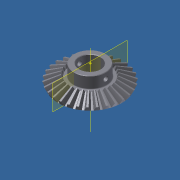
# Autodesk Inventor part: Bevel Gear1
Saved by Autodesk Inventor 2012 SP2 (Build 160219200, 219)
## iProperties
Created: 2012-07-24
Part Number: Bevel Gear1
Material: Steel, Mild
Document SubType Name: Modeling
Designer: bruno.silveira
Categories: <?xml version="1.0" encoding="UTF-16"?> <MemberInstance><Categories><FamilyTemplate><FamilyTemplateParameter ValueType="xs:double" Id="1" ObjectReferenceKey="da_z" ObjectType="kUserParameterObject"/><FamilyTemplateParameter ValueType="xs:double" Id="2" ObjectReferenceKey="da_b" ObjectType="kUserParameterObject"/><FamilyTemplateParameter ValueType="xs:double" Id="3" ObjectReferenceKey="da_beta" ObjectType="kUserParameterObject"/><FamilyTemplateParameter ValueType="xs:double" Id="4" ObjectReferenceKey="da_dae" ObjectType="kUserParameterObject"/><FamilyTemplateParameter ValueType="xs:double" Id="5" ObjectReferenceKey="da_ve" ObjectType="kUserParameterObject"/><FamilyTemplateParameter ValueType="xs:double" Id="6" ObjectReferenceKey="da_omega" ObjectType="kUserParameterObject"/><FamilyTemplateParameter ValueType="xs:string" Id="7" ObjectReferenceKey="EAIAABAAAAAAHwAAAAAAAIAAAAAAAAAA" ObjectType="83914240" SubObjectId="SurfaceGeometry"/></FamilyTemplate><ParamToTemplateMap><ParamToTemplate CategoryParameter="//CategoryParameter[@InternalName='046C89C9-8512-4d59-83FE-43B91F4F132A']" TemplateParameter="1"/><ParamToTemplate CategoryParameter="//CategoryParameter[@InternalName='2552DF32-E462-4b46-AEBF-C6C7768E72AC']" TemplateParameter="2"/><ParamToTemplate CategoryParameter="//CategoryParameter[@InternalName='C9EE641D-15FC-4fae-A226-E94C4372FDD7']" TemplateParameter="3"/><ParamToTemplate><ParamToTemplate CategoryParameter="//CategoryParameter[@InternalName='00B6519A-459B-49c7-AD84-2E56D39A5744']" ConstantValue="0.000000"/></ParamToTemplate><ParamToTemplate><ParamToTemplate CategoryParameter="//CategoryParameter[@InternalName='04B31F0E-C7A6-4894-AA32-9629BEFACF47']" ConstantValue="1.000000"/></ParamToTemplate><ParamToTemplate><ParamToTemplate CategoryParameter="//CategoryParameter[@InternalName='43CBEC2E-7847-49e7-A936-2F7889FCB2D9']" ConstantValue="0.200000"/></ParamToTemplate><ParamToTemplate><ParamToTemplate CategoryParameter="//CategoryParameter[@InternalName='B1EFC894-105D-4ebd-86BF-FA20ED196853']" ConstantValue="0.300000"/></ParamToTemplate><ParamToTemplate><ParamToTemplate CategoryParameter="//CategoryParameter[@InternalName='51175063-3D10-4879-93E8-6246FE8B403D']" ConstantValue="2060000000.000000"/></ParamToTemplate><ParamToTemplate><ParamToTemplate CategoryParameter="//CategoryParameter[@InternalName='A3A52E27-4454-46a9-B0BD-C932399B70AF']" ConstantValue="0.300000"/></ParamToTemplate><ParamToTemplate CategoryParameter="//CategoryParameter[@InternalName='2A200944-5A8C-41ca-B96E-8520D2E510F1']" TemplateParameter="4"/><ParamToTemplate><ParamToTemplate CategoryParameter="//CategoryParameter[@InternalName='1A637F62-92C8-44bc-B81F-10802510B579']" ConstantValue="2.791976"/></ParamToTemplate><ParamToTemplate CategoryParameter="//CategoryParameter[@InternalName='B52DD4BE-6863-48fb-BF58-89EF6F9EC65C']" TemplateParameter="5"/><ParamToTemplate><ParamToTemplate CategoryParameter="//CategoryParameter[@InternalName='3956BFF2-84D2-457d-93C2-9B0613DEBA67']" ConstantValue="0.596956"/></ParamToTemplate><ParamToTemplate CategoryParameter="//CategoryParameter[@InternalName='739CFA02-461B-4bf8-8049-181FCAD8B28F']" TemplateParameter="6"/><ParamToTemplate><ParamToTemplate CategoryParameter="//CategoryParameter[@InternalName='A27E999F-E2CE-4481-8A2A-EBF499C4C3C5']" ConstantValue="0.000000"/></ParamToTemplate><ParamToTemplate><ParamToTemplate CategoryParameter="//CategoryParameter[@InternalName='9E1B4470-B2D3-4ff1-B813-535BB4CDF51A']" ConstantValue="3520000.000000"/></ParamToTemplate><ParamToTemplate><ParamToTemplate CategoryParameter="//CategoryParameter[@InternalName='F8452263-BFF6-458c-9FB1-07C4B99E95CD']" ConstantValue="11400000.000000"/></ParamToTemplate><ParamToTemplate><ParamToTemplate CategoryParameter="//CategoryParameter[@InternalName='3E3BB259-FD49-497f-8171-6EBC954A3479']" ConstantValue="2.000000"/></ParamToTemplate><ParamToTemplate CategoryParameter="//CategoryParameter[@InternalName='27C3BAF2-7550-4e4b-AE2C-0DB134B7D9B7']" TemplateParameter="7"/></ParamToTemplateMap><Category DisplayName="Gear" InternalName="DC85795E-93AB-48d5-8EEE-5A27447B64BD" Mnemonic="Gear"><CategoryParameter DisplayName="z" InternalName="046C89C9-8512-4d59-83FE-43B91F4F132A" Mnemonic="z"/><CategoryParameter DisplayName="b" InternalName="2552DF32-E462-4b46-AEBF-C6C7768E72AC" Mnemonic="b"/><CategoryParameter DisplayName="||b|" InternalName="C9EE641D-15FC-4fae-A226-E94C4372FDD7" Mnemonic="beta"/><CategoryParameter DisplayName="x" InternalName="00B6519A-459B-49c7-AD84-2E56D39A5744" Mnemonic="x"/><CategoryParameter DisplayName="a*" InternalName="04B31F0E-C7A6-4894-AA32-9629BEFACF47" Mnemonic="a"/><CategoryParameter DisplayName="c*" InternalName="43CBEC2E-7847-49e7-A936-2F7889FCB2D9" Mnemonic="c"/><CategoryParameter DisplayName="r|.f|*" InternalName="B1EFC894-105D-4ebd-86BF-FA20ED196853" Mnemonic="rf"/><CategoryParameter DisplayName="E" InternalName="51175063-3D10-4879-93E8-6246FE8B403D" Mnemonic="E"/><CategoryParameter DisplayName="||m|" InternalName="A3A52E27-4454-46a9-B0BD-C932399B70AF" Mnemonic="mi"/><Category DisplayName="BevelGear" InternalName="0C98F69A-0C2B-4791-B2FE-7691BB227E77" Mnemonic="BevelGear"><CategoryParameter DisplayName="d|.ae|" InternalName="2A200944-5A8C-41ca-B96E-8520D2E510F1" Mnemonic="dae"/><CategoryParameter DisplayName="d|.ai|" InternalName="1A637F62-92C8-44bc-B81F-10802510B579" Mnemonic="dai"/><CategoryParameter DisplayName="A|.e|" InternalName="B52DD4BE-6863-48fb-BF58-89EF6F9EC65C" Mnemonic="ve"/><CategoryParameter DisplayName="A|.i|" InternalName="3956BFF2-84D2-457d-93C2-9B0613DEBA67" Mnemonic="vi"/><CategoryParameter DisplayName="||S|" InternalName="739CFA02-461B-4bf8-8049-181FCAD8B28F" Mnemonic="omega"/><CategoryParameter DisplayName="x|.t|" InternalName="A27E999F-E2CE-4481-8A2A-EBF499C4C3C5" Mnemonic="xt"/><CategoryParameter DisplayName="||s||.Flim|" InternalName="9E1B4470-B2D3-4ff1-B813-535BB4CDF51A" Mnemonic="sFlim"/><CategoryParameter DisplayName="||s||.Hlim|" InternalName="F8452263-BFF6-458c-9FB1-07C4B99E95CD" Mnemonic="sHlim"/><CategoryParameter DisplayName="type" InternalName="3E3BB259-FD49-497f-8171-6EBC954A3479" Mnemonic="type"/><CategoryParameter DisplayName="PitchDiameter" InternalName="27C3BAF2-7550-4e4b-AE2C-0DB134B7D9B7" Mnemonic="IDS_PITCHDIAM"/></Category></Category></Categories></MemberInstance>
Mass: 60.9118 g
Surface Area: 34.3074 cm^2
Volume: 7.7496 cm^3
Density: 7.86 g/cm^3
CustomPartVersion: 1
Author: bruno.silveira
Autodesk Inventor part; units mm, degrees
ref_plane "Mesh Plane2" through (0, 0, 0) normal (0.9945219, 0.1045285, 0) x (0, 0, 1)
sketch "Teeth Body Sketch" plane through (0, 0, 0) normal (1, 0, 0) x (0, 1, 0)
  line L0 (0, 0) -> (21.695016, -12.859969) construction
  line L1 (21.695016, -12.859969) -> (23.17082, -9.908359)
  line L2 (23.17082, -9.908359) -> (0, 0) construction
  line L3 (22.5, -11.25) -> (0, 0) construction
  line L4 (13.070744, -7.747833) -> (13.959882, -5.969557)
  line L5 (21.695016, -12.859969) -> (13.070744, -7.747833)
  line L6 (23.17082, -9.908359) -> (13.959882, -5.969557)
  line L7 (0, -39.386751) -> (0, 6.564458)
  line L8 (0, -11.25) -> (23.17082, -11.25) construction
  dimension "d0" = 45
  dimension "d1" = 43.39003
  dimension "d2" = 46.34164
  dimension "d3" = 10
  dimension "d4" = 9.90836
  constraints: 16 end point, 4 point on line, 3 perpendicular, 2 collinear, 1 horizontal alignment, 1 vertical alignment
  measures "d0" diameter of L3.start L7
  measures "d1" diameter of L0.end L7
  measures "d2" diameter of L1.end L7
  measures "d3" distance between parallel lines of L1 L4
  measures "d4" vertical distance of L1.end L0.start
revolve "Teeth Body" add sketch "Teeth Body Sketch" angle 360 about axis through (0, 0, 0) along (0, 0, 1)
ref_plane "Tooth Plane" through (0, 22.5, -11.25) normal (0, -0.8944272, 0.4472136) x (1, 0, 0)
sketch "Start Sketch" plane through (0, 22.5, -11.25) normal (0, -0.8944272, 0.4472136) x (1, 0, 0)
  line L0 (0, -23.505131) -> (0, 10.644758)
  arc A0 (-0.514983, -2.196) -> (-2.349882, 2.437684) centre (-17.750519, -6.340979) ccw
  arc A1 (2.349882, 2.437684) -> (0.514983, -2.196) centre (17.750519, -6.340979) ccw
  line L1 (-0.514983, -2.196) -> (0.514983, -2.196)
  arc A2 (2.349882, 2.437684) -> (-2.349882, 2.437684) centre (0, -50.311529) ccw
  dimension "d7" = 17.72694
  dimension "d8" = 17.75052
  dimension "d9" = 43.97055
  dimension "d57" = 52.80153
  dimension "d58" = 48.11553
  constraints: 6 point on circle, 3 centre point, 3 symmetric about line, 2 end point, 1 coincident, 1 perpendicular, 1 other
  measures "d7" radius of A0
  measures "d8" horizontal distance of point (0, -50.312) A0.centre
  measures "d9" vertical distance of point (0, -50.312) A0.centre
  measures "d57" radius of A2
  measures "d58" distance from line of A2.centre L1
sketch "End Sketch" plane through (0, 13.408148, -6.704074) normal (0, -0.8944272, 0.4472136) x (1, 0, 0)
  line L0 (0, -15.358918) -> (0, 6.982715)
  arc A0 (-0.307403, -1.26052) -> (-1.402686, 1.505408) centre (-10.595599, -3.734731) ccw
  arc A1 (1.402686, 1.505408) -> (0.307403, -1.26052) centre (10.595599, -3.734731) ccw
  line L1 (-0.307403, -1.26052) -> (0.307403, -1.26052)
  arc A2 (1.402686, 1.505408) -> (-1.402686, 1.505408) centre (0, -29.981529) ccw
  dimension "d12" = 10.58153
  dimension "d15" = 10.5956
  dimension "d16" = 26.2468
  dimension "d59" = 31.51817
  dimension "d60" = 28.72101
  constraints: 6 point on circle, 3 centre point, 3 symmetric about line, 2 end point, 1 coincident, 1 other
  measures "d12" radius of A0
  measures "d15" horizontal distance of A0.centre point (0, -29.982)
  measures "d16" vertical distance of A0.centre point (0, -29.982)
  measures "d59" radius of A2
  measures "d60" distance from line of A2.centre L1
loft "Loft" cut profiles "Start Sketch", "End Sketch"
pattern_circular "Circular Pattern" count 30 over 360 about axis through (0, 0, 0) along (0, 0, 1) of "Loft"
ref_plane "End Plane" through (0, 13.408148, -6.704074) normal (0, -0.8944272, 0.4472136) x (1, 0, 0)
sketch3d "3D Sketch Right"
ref_plane "End Plane Right" through (-2.732404, 13.126781, -6.704074) normal (0.1822725, -0.8756579, 0.4472136) x (0.9790153, 0.2037868, 0)
sketch "End Sketch Right" plane through (-2.732404, 13.126781, -6.704074) normal (0.1822725, -0.8756579, 0.4472136) x (0.9790153, 0.2037868, 0)
  arc A0 (-0.307403, -1.26052) -> (-1.402686, 1.505408) centre (-10.595599, -3.734731) ccw
  line L0 (0, -38.384553) -> (0, 12.194071)
  arc A1 (1.402686, 1.505408) -> (0.307403, -1.26052) centre (10.595599, -3.734731) ccw
  line L1 (-0.307403, -1.26052) -> (0.307403, -1.26052)
  arc A2 (1.402686, 1.505408) -> (-1.402686, 1.505408) centre (0, -29.981529) ccw
  dimension "d70" = 10.5956
  dimension "d71" = 26.2468
  dimension "d72" = 10.58153
  dimension "d73" = 28.72101
  dimension "d74" = 31.51817
  constraints: 6 point on circle, 3 centre point, 3 symmetric about line, 2 end point, 1 coincident, 1 perpendicular, 1 other
  measures "d70" horizontal distance of A2.centre A0.centre
  measures "d71" vertical distance of point (0, -29.982) A0.centre
  measures "d72" radius of A0
  measures "d73" distance from line of point (0, -29.982) L1
  measures "d74" radius of A2
feature "Loft Right" [suppressed]
pattern_circular "Circular Pattern Right" [suppressed]
sketch3d "3D Sketch Left"
ref_plane "End Plane Left" through (2.802075, 13.126781, -6.746684) normal (-0.1865226, -0.8737959, 0.4490991) x (0.9779671, -0.2087592, 0)
sketch "End Sketch Left" plane through (2.802075, 13.126781, -6.746684) normal (-0.1865226, -0.8737959, 0.4490991) x (0.9779671, -0.2087592, 0)
  line L0 (0, -40.074202) -> (0, 13.91771)
  arc A0 (-0.307403, -1.228836) -> (-1.402686, 1.537093) centre (-10.595599, -3.703047) ccw
  arc A1 (1.402686, 1.537093) -> (0.307403, -1.228836) centre (10.595599, -3.703047) ccw
  line L1 (-0.307403, -1.228836) -> (0.307403, -1.228836)
  ellipse E0 centre (0, -5.333691) end of major axis (13.959882, -5.333691) minor radius 6.26937
  arc A2 (1.402686, 1.537093) -> (-1.402686, 1.537093) centre (0, -29.949845) ccw
  dimension "d56" = 6.26937
  dimension "d30" = 10.58153
  dimension "d31" = 10.5956
  dimension "d32" = 26.2468
  dimension "d61" = 31.51817
  dimension "d62" = 28.72101
  constraints: 6 point on circle, 3 centre point, 3 symmetric about line, 2 end point, 1 coincident, 2 other
  measures "d30" radius of A0
  measures "d31" horizontal distance of point (0, -29.95) A0.centre
  measures "d32" vertical distance of A0.centre point (0, -29.95)
  measures "d61" radius of A2
  measures "d62" distance from line of point (0, -29.95) L1
feature "Loft Left" [suppressed]
pattern_circular "Circular Pattern Left" [suppressed]
sketch "Body Sketch" plane through (0, 0, 0) normal (1, 0, 0) x (0, 1, 0)
  line L0 (0, -35.037536) -> (0, -19.530831)
  line L1 (21.695016, -12.859969) -> (13.070744, -7.747833)
  line L2 (13.070744, -7.747833) -> (0, -7.747833)
  line L3 (21.695016, -12.859969) -> (0, -12.859969)
  constraints: 4 end point, 2 perpendicular, 2 point on line
sketch "Body Sketch outline for Fix Body" plane through (0, 0, 0) normal (1, 0, 0) x (0, 1, 0)
  line L0 (0, -12.859969) -> (21.695016, -12.859969)
  line L1 (0, -7.747833) -> (0, -12.859969)
  line L2 (13.070744, -7.747833) -> (0, -7.747833)
  line L3 (21.695016, -12.859969) -> (13.070744, -7.747833)
revolve "Fix Body" add sketch "Body Sketch outline for Fix Body" angle 360 about axis through (0, 0, 0) along (0, 0, 1)
sketch "Sketch6" plane through (0, 0, 0) normal (1, 0, 0) x (0, 1, 0)
  line L0 (22.5, -11.25) -> (0, 0)
  line L1 (0, -37.799919) -> (0, 6.299986)
surface revolve "Pitch Diameter" sketch "Sketch6" angle 360 about axis through (0, 0, 0) along (0, 0, 1) shown no curves L0
sketch "Sketch8" plane through (0, 0, -12.859969) normal (0, 0, -1) x (-1, 0, 0)
  arc A0 (3.90857, 21.340028) -> (0.613682, 21.686334) centre (0, 0) ccw
  circle A1 centre (0, 0) radius 11
  dimension "d94" = 22
  constraints: 1 centre point, 1 coincident
  measures "d94" diameter of A1
extrude "Extrusion1" add sketch "Sketch8" along normal blind 2.5
sketch "Sketch9" plane through (0, 0, -7.747833) normal (0, 0, 1) x (1, 0, 0)
  arc A0 (2.366492, 12.854729) -> (0.35787, 13.065844) centre (0, 0) ccw
  circle A1 centre (0, 0) radius 11
  dimension "d97" = 22
  constraints: 1 centre point, 1 coincident
  measures "d97" diameter of A1
extrude "Extrusion2" add sketch "Sketch9" along normal blind 8
sketch "Sketch10" plane through (0, 0, -15.359969) normal (0, 0, -1) x (-1, 0, 0)
  circle A0 centre (0, 0) radius 11 projected
  circle A1 centre (0, 0) radius 7.25
  dimension "d100" = 14.5
  constraints: 1 centre point, 1 coincident
  measures "d100" diameter of A1
extrude "Extrusion3" cut sketch "Sketch10" against normal blind 20 contours A1
chamfer "Chamfer1" distance 0.3 angle 45 4 edges at (7.25, 0, 0.2522) (-11, 0, 0.2522) (11, 0, -15.36) (7.25, 0, -15.36)
fillet "Fillet1" radius 0.5 2 edges at (11, 0, -12.86) (-11, 0, -7.7478)
sketch "Sketch11" plane through (0, 0, 0) normal (1, 0, 0) x (0, 1, 0)
  circle A0 centre (0, -3.747833) radius 1.5875
  line L0 (-10.7, 0.252167) -> (10.7, 0.252167)
  point P0 (0, 0)
  dimension "d107" = 3.175
  dimension "d108" = 4
  constraints: 1 centre point
  measures "d107" diameter of A0
  measures "d108" distance from line of L0 A0.centre
extrude "Extrusion4" cut sketch "Sketch11" along normal mid plane 25
equation "\"d0\" = da_de"
equation "\"d1\" = da_dfe"
equation "\"d2\" = da_dae"
equation "\"d3\" = da_b"
equation "\"d4\" = da_ve"
equation "\"d7\" = fd_rr"
equation "\"d8\" = fd_x"
equation "\"d9\" = fd_y"
equation "\"d57\" = 0.5 * fd_dva + 0.3 * da_he"
equation "\"d58\" = 0.5 * fd_dva - 1.12 * da_he"
equation "\"da_teethtype\" = 0"
equation "\"da_b\" = 10"
equation "\"da_de\" = 45"
equation "\"da_dae\" = 46.34164"
equation "\"da_dfe\" = 43.39003"
equation "\"da_le\" = 25.15576"
equation "\"da_omega\" = 90deg"
equation "\"da_beta\" = 0"
equation "\"da_delta\" = 63.434949deg"
equation "\"da_alpha\" = 20deg"
equation "\"da_he\" = 3.3"
equation "\"da_ve\" = 9.90836"
equation "\"da_zv\" = 67.082039"
equation "\"fd_loft\" = da_b + 0.05 * da_he"
equation "\"fd_x\" = fd_x1 + fd_x2"
equation "\"fd_y\" = fd_y1 - fd_y2"
equation "\"fd_dd\" = fd_dva - 0.8 * da_he"
equation "\"da_dvw\" = 100.62306"
equation "\"d11\" = fd_loft"
equation "\"da_dm\" = 36.05573"
equation "\"da_x\" = 0"
equation "\"da_m\" = 1.5"
equation "\"d50\" = da_omega"
equation "\"fd_rr\" = 17.726944"
equation "\"fd_dva\" = 103.623059"
equation "\"fd_x1\" = 1.191076"
equation "\"fd_x2\" = 16.559443"
equation "\"fd_y1\" = 50.297429"
equation "\"fd_y2\" = 6.326879"
body "Solid1"
body "Srf1"
